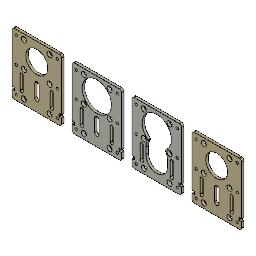
Master Panels v19 (Autodesk Fusion 360 design; units mm, degrees)
Autodesk Fusion 360 part; units mm, degrees
note: some values were not read from the file. Set by a fixed rule: which sketch regions a step uses.
sketch "Sketch1" plane through (0, 0, 0) normal (0, 0, 1) x (1, 0, 0)
  line L0 (-75, 0) -> (75, 0) construction
  line L1 (0, 75) -> (0, -100) construction
  line L2 (0, -100) -> (0, -250) construction
  circle A0 centre (0, 0) radius 12.7
  line L3 (0, 0) -> (-53.033, 53.033) construction
  line L4 (0, 0) -> (75, 0) construction
  circle A1 centre (-15, 15) radius 2.95
  circle A2 centre (15, 15) radius 2.95
  circle A3 centre (-15, -15) radius 2.95
  circle A4 centre (15, -15) radius 2.95
  circle A5 centre (-24, 15) radius 1.4
  circle A6 centre (24, 15) radius 1.4
  circle A7 centre (-24, -15) radius 1.4
  circle A8 centre (24, -15) radius 1.4
  circle A9 centre (-24, -45) radius 1.4
  circle A10 centre (24, -45) radius 1.4
  line L5 (-29, 21) -> (29, 21)
  line L6 (29, 21) -> (29, -51)
  line L7 (29, -51) -> (-29, -51)
  line L8 (-29, -51) -> (-29, 21)
  circle A11 centre (-15, -45) radius 2.95
  circle A12 centre (15, -45) radius 2.95
  line L9 (15.75, -21.7504) -> (15.75, -38.25)
  arc A13 (15.75, -38.25) -> (19.25, -38.25) centre (17.5, -38.25) ccw
  line L10 (19.25, -38.25) -> (19.25, -21.7504)
  arc A14 (19.25, -21.7504) -> (15.75, -21.7504) centre (17.5, -21.7504) ccw
  line L11 (17.5, -20.0004) -> (17.5, -40) construction
  line L12 (-17.5, -20.0004) -> (-17.5, -40) construction
  line L13 (-15.75, -21.7504) -> (-15.75, -38.25)
  arc A15 (-15.75, -21.7504) -> (-19.25, -21.7504) centre (-17.5, -21.7504) ccw
  line L14 (-19.25, -38.25) -> (-19.25, -21.7504)
  arc A16 (-19.25, -38.25) -> (-15.75, -38.25) centre (-17.5, -38.25) ccw
  line L15 (-2.5, -22.5004) -> (-2.5, -37.5)
  arc A17 (-2.5, -37.5) -> (2.5, -37.5) centre (0, -37.5) ccw
  line L16 (2.5, -37.5) -> (2.5, -22.5004)
  arc A18 (2.5, -22.5004) -> (-2.5, -22.5004) centre (0, -22.5004) ccw
  line L17 (0, -20.0004) -> (0, -40) construction
  line L18 (-29, -51) -> (-26, -51)
  line L19 (-26, -51) -> (-26, -39.1)
  line L20 (-26, -39.1) -> (-29, -39.1)
  line L21 (-29, -39.1) -> (-29, -51)
  line L22 (-29, -42) -> (-26, -42)
  line L23 (29, -42) -> (26, -42)
  line L24 (26, -51) -> (26, -39.1)
  line L25 (26, -39.1) -> (29, -39.1)
  dimension "d1" = 25.4
  dimension "d2" = 135
  dimension "d3" = 75
  dimension "d4" = 5.9
  dimension "d5" = 15
  dimension "d8" = 30
  dimension "d9" = -60
  dimension "d10" = 2.8
  dimension "d11" = 9
  dimension "d14" = 48
  dimension "d15" = -60
  dimension "d16" = 5
  dimension "d17" = 6
  dimension "d18" = 5
  dimension "d19" = 6
  dimension "d20" = 3.5
  dimension "d21" = 17.5
  dimension "d22" = 5
  dimension "d38" = 58
  dimension "d39" = 72
  dimension "d42" = 3
  dimension "d43" = 11.9
  dimension "d44" = 9
  measures "d1" diameter of A0
  measures "d2" angle of L3 L4
  measures "d3" distance of A0.centre L3.end
  measures "d4" diameter of A1
  measures "d5" distance of L0 A1.centre
  measures "d10" diameter of A5
  measures "d11" distance of A1.centre A5.centre
  measures "d16" distance of A6.centre L6
  measures "d17" distance of A2.centre L5
  measures "d18" distance of A9.centre L8
  measures "d19" distance of L7 A11.centre
  measures "d20" diameter of A13
  measures "d21" distance of L1 L11
  measures "d22" diameter of A17
  measures "d38" distance of L6.end L7.end
  measures "d39" distance of L5.end L6.end
  measures "d42" distance of L7.end L18.end
  measures "d43" distance of L7.end L20.end
  measures "d44" distance of L7 L22
extrude "Extrude1" add sketch "Sketch1" along normal blind 3 contours L5 L6 L7 L8 L19 L20 L24 L25 | L7 L8 L18 L19 L21 L22 | L6 L7 L23 L24 makes body 1
fillet "Fillet1" radius 2.5 4 edges at (-29, 21, 1.5) (29, 21, 1.5) (29, -51, 1.5) (-29, -51, 1.5) on bodies 1
ref_plane "WorkPlane1" through (0, -15, 3) normal (0, 0, 1) x (1, 0, 0)
sketch "Sketch2" plane through (0, -15, 3) normal (0, 0, 1) x (1, 0, 0)
  arc A0 (-29, -33.5) -> (-26.5, -36) centre (-26.5, -33.5) ccw
  line L0 (-26.5, -36) -> (26.5, -36)
  arc A1 (26.5, -36) -> (29, -33.5) centre (26.5, -33.5) ccw
  line L1 (29, -33.5) -> (29, -27)
  arc A2 (29, 33.5) -> (26.5, 36) centre (26.5, 33.5) ccw
  line L2 (26.5, 36) -> (-26.5, 36)
  arc A3 (-26.5, 36) -> (-29, 33.5) centre (-26.5, 33.5) ccw
  line L3 (-29, 33.5) -> (-29, -24.1)
  arc A4 (19.25, -6.7504) -> (15.75, -6.7504) centre (17.5, -6.7504) ccw
  line L4 (19.25, -6.7504) -> (19.25, -23.25)
  arc A5 (15.75, -23.25) -> (19.25, -23.25) centre (17.5, -23.25) ccw
  line L5 (15.75, -23.25) -> (15.75, -6.7504)
  arc A6 (-15.75, -6.7504) -> (-19.25, -6.7504) centre (-17.5, -6.7504) ccw
  line L6 (-15.75, -6.7504) -> (-15.75, -23.25)
  arc A7 (-19.25, -23.25) -> (-15.75, -23.25) centre (-17.5, -23.25) ccw
  line L7 (-19.25, -23.25) -> (-19.25, -6.7504)
  circle A8 centre (15, -30) radius 2.95
  arc A9 (2.5, -7.5004) -> (-2.5, -7.5004) centre (0, -7.5004) ccw
  line L8 (2.5, -7.5004) -> (2.5, -22.5)
  arc A10 (-2.5, -22.5) -> (2.5, -22.5) centre (0, -22.5) ccw
  line L9 (-2.5, -22.5) -> (-2.5, -7.5004)
  circle A11 centre (24, -30) radius 1.4
  circle A12 centre (-15, -30) radius 2.95
  circle A13 centre (-24, -30) radius 1.4
  circle A14 centre (24, 0) radius 1.4
  circle A15 centre (-24, 0) radius 1.4
  circle A16 centre (24, 30) radius 1.4
  circle A17 centre (-24, 30) radius 1.4
  circle A18 centre (15, 0) radius 2.95
  circle A19 centre (-15, 0) radius 2.95
  circle A20 centre (15, 30) radius 2.95
  circle A21 centre (-15, 30) radius 2.95
  circle A22 centre (0, 15) radius 12.7
  circle A23 centre (0, 15) radius 16.95
  line L10 (29, -27) -> (26, -27)
  line L11 (26, -27) -> (26, -24.1)
  line L12 (26, -24.1) -> (29, -24.1)
  line L13 (29, -24.1) -> (29, 33.5)
  line L14 (-29, -24.1) -> (-26, -24.1)
  line L15 (-26, -24.1) -> (-26, -27)
  line L16 (-26, -27) -> (-29, -27)
  line L17 (-29, -27) -> (-29, -33.5)
  dimension "d27" = 33.9
  measures "d27" diameter of A23
extrude "Extrude2" add sketch "Sketch2" against normal blind 3 separate body contours A0 L0 A1 L1 A2 L2 A3 L3 L10 L11 L12 L13 L14 L15 L16 L17 makes body 2
ref_plane "WorkPlane2" through (0, -15, 3) normal (0, 0, 1) x (1, 0, 0)
sketch "Sketch3" plane through (0, -15, 3) normal (0, 0, 1) x (1, 0, 0)
  arc A0 (-29, -33.5) -> (-26.5, -36) centre (-26.5, -33.5) ccw
  line L0 (-26.5, -36) -> (26.5, -36)
  arc A1 (26.5, -36) -> (29, -33.5) centre (26.5, -33.5) ccw
  line L1 (29, -33.5) -> (29, -27)
  arc A2 (29, 33.5) -> (26.5, 36) centre (26.5, 33.5) ccw
  line L2 (26.5, 36) -> (-26.5, 36)
  arc A3 (-26.5, 36) -> (-29, 33.5) centre (-26.5, 33.5) ccw
  line L3 (-29, 33.5) -> (-29, -24.1)
  arc A4 (19.25, -6.7504) -> (15.75, -6.7504) centre (17.5, -6.7504) ccw
  line L4 (19.25, -6.7504) -> (19.25, -23.25)
  arc A5 (15.75, -23.25) -> (19.25, -23.25) centre (17.5, -23.25) ccw
  line L5 (15.75, -23.25) -> (15.75, -6.7504)
  arc A6 (-15.75, -6.7504) -> (-19.25, -6.7504) centre (-17.5, -6.7504) ccw
  line L6 (-15.75, -6.7504) -> (-15.75, -23.25)
  arc A7 (-19.25, -23.25) -> (-15.75, -23.25) centre (-17.5, -23.25) ccw
  line L7 (-19.25, -23.25) -> (-19.25, -6.7504)
  circle A8 centre (15, -30) radius 2.95
  arc A9 (2.5, -7.5004) -> (-2.5, -7.5004) centre (0, -7.5004) ccw
  line L8 (2.5, -7.5004) -> (2.5, -22.5)
  arc A10 (-2.5, -22.5) -> (2.5, -22.5) centre (0, -22.5) ccw
  line L9 (-2.5, -22.5) -> (-2.5, -7.5004)
  circle A11 centre (24, -30) radius 1.4
  circle A12 centre (-15, -30) radius 2.95
  circle A13 centre (-24, -30) radius 1.4
  circle A14 centre (24, 0) radius 1.4
  circle A15 centre (-24, 0) radius 1.4
  circle A16 centre (24, 30) radius 1.4
  circle A17 centre (-24, 30) radius 1.4
  circle A18 centre (15, 0) radius 2.95
  circle A19 centre (-15, 0) radius 2.95
  circle A20 centre (15, 30) radius 2.95
  circle A21 centre (-15, 30) radius 2.95
  circle A22 centre (0, 15) radius 12.7
  circle A23 centre (0, 15) radius 16.95
  line L10 (12.5, -15) -> (12.5, -7.5004)
  arc A24 (12.5, -7.5004) -> (-12.5, -7.5004) centre (0, -7.5004) ccw
  line L11 (-12.5, -7.5004) -> (-12.5, -15)
  arc A25 (-12.5, -15) -> (12.5, -15) centre (0, -15) ccw
  line L12 (0, -15) -> (0, -7.5004) construction
  line L13 (10, -7.5004) -> (-10, -7.5004)
  line L14 (-10, -7.5004) -> (-10, 7.5004)
  line L15 (-10, 7.5004) -> (10, 7.5004)
  line L16 (10, 7.5004) -> (10, -7.5004)
  line L17 (10, -7.5004) -> (-10, 7.5004) construction
  line L18 (-10, -7.5004) -> (10, 7.5004) construction
  line L19 (29, -27) -> (26, -27)
  line L20 (26, -27) -> (26, -24.1)
  line L21 (26, -24.1) -> (29, -24.1)
  line L22 (29, -24.1) -> (29, 33.5)
  line L23 (-29, -24.1) -> (-26, -24.1)
  line L24 (-26, -24.1) -> (-26, -27)
  line L25 (-26, -27) -> (-29, -27)
  line L26 (-29, -27) -> (-29, -33.5)
  dimension "d31" = 25
  dimension "d32" = 20
  measures "d31" diameter of A24
  measures "d32" distance of L14.end L15.end
extrude "Extrude3" add sketch "Sketch3" against normal blind 3 separate body makes body 3
ref_plane "WorkPlane3" through (0, -15, 3) normal (0, 0, 1) x (1, 0, 0)
sketch "Sketch4" plane through (0, -15, 3) normal (0, 0, 1) x (1, 0, 0)
  arc A0 (-29, -33.5) -> (-26.5, -36) centre (-26.5, -33.5) ccw
  line L0 (-26.5, -36) -> (26.5, -36)
  arc A1 (26.5, -36) -> (29, -33.5) centre (26.5, -33.5) ccw
  line L1 (29, -33.5) -> (29, -27)
  arc A2 (29, 33.5) -> (26.5, 36) centre (26.5, 33.5) ccw
  line L2 (26.5, 36) -> (-26.5, 36)
  arc A3 (-26.5, 36) -> (-29, 33.5) centre (-26.5, 33.5) ccw
  line L3 (-29, 33.5) -> (-29, -24.1)
  arc A4 (19.25, -6.7504) -> (15.75, -6.7504) centre (17.5, -6.7504) ccw
  line L4 (19.25, -6.7504) -> (19.25, -23.25)
  arc A5 (15.75, -23.25) -> (19.25, -23.25) centre (17.5, -23.25) ccw
  line L5 (15.75, -23.25) -> (15.75, -6.7504)
  arc A6 (-15.75, -6.7504) -> (-19.25, -6.7504) centre (-17.5, -6.7504) ccw
  line L6 (-15.75, -6.7504) -> (-15.75, -23.25)
  arc A7 (-19.25, -23.25) -> (-15.75, -23.25) centre (-17.5, -23.25) ccw
  line L7 (-19.25, -23.25) -> (-19.25, -6.7504)
  circle A8 centre (15, -30) radius 2.95
  arc A9 (2.5, -7.5004) -> (-2.5, -7.5004) centre (0, -7.5004) ccw
  line L8 (2.5, -7.5004) -> (2.5, -22.5)
  arc A10 (-2.5, -22.5) -> (2.5, -22.5) centre (0, -22.5) ccw
  line L9 (-2.5, -22.5) -> (-2.5, -7.5004)
  circle A11 centre (24, -30) radius 1.4
  circle A12 centre (-15, -30) radius 2.95
  circle A13 centre (-24, -30) radius 1.4
  circle A14 centre (24, 0) radius 1.4
  circle A15 centre (-24, 0) radius 1.4
  circle A16 centre (24, 30) radius 1.4
  circle A17 centre (-24, 30) radius 1.4
  circle A18 centre (15, 0) radius 2.95
  circle A19 centre (-15, 0) radius 2.95
  circle A20 centre (15, 30) radius 2.95
  circle A21 centre (-15, 30) radius 2.95
  circle A22 centre (0, 15) radius 12.7
  line L10 (29, -27) -> (26, -27)
  line L11 (26, -27) -> (26, -24.1)
  line L12 (26, -24.1) -> (29, -24.1)
  line L13 (29, -24.1) -> (29, 33.5)
  line L14 (-29, -24.1) -> (-26, -24.1)
  line L15 (-26, -24.1) -> (-26, -27)
  line L16 (-26, -27) -> (-29, -27)
  line L17 (-29, -27) -> (-29, -33.5)
extrude "Extrude4" add sketch "Sketch4" against normal blind 3 separate body makes body 4
copy_body "Body->Comp1" bodies 4 removing the originals makes body 5 in component "Component"
copy_body "Body->Comp2" bodies 3 removing the originals makes body 6 in component "Component'"
copy_body "Body->Comp3" bodies 2 removing the originals makes body 7 in component "Component''"
copy_body "Body->Comp4" bodies 1 removing the originals makes body 8 in component "Component'''"
copy_body "Body->Comp1'" bodies 5 removing the originals makes body 9 in component "Component''''"
copy_body "Body->Comp1''" bodies 6 removing the originals makes body 10 in component "Component'''''"
copy_body "Body->Comp1'''" bodies 7 removing the originals makes body 11 in component "Component''''''"
copy_body "Body->Comp1''''" bodies 8 removing the originals makes body 12 in component "Component'''''''"
move_body "Move2" bodies 11 to x (1, 0, 0) y (0, 1, 0) z (0, 0, 1) at (70, 0, 0) in component "Component''''''"
move_body "Move2'" bodies 10 to x (1, 0, 0) y (0, 1, 0) z (0, 0, 1) at (140, 0, 0) in component "Component'''''"
move_body "Move1" bodies 9 to x (1, 0, 0) y (0, 1, 0) z (0, 0, 1) at (210, 0, 0) in component "Component''''"
component "Component" placed x (1, 0, 0) y (0, 1, 0) z (0, 0, 1) at (0, 0, 0)
component "Component'" placed x (1, 0, 0) y (0, 1, 0) z (0, 0, 1) at (0, 0, 0)
component "Component''" placed x (1, 0, 0) y (0, 1, 0) z (0, 0, 1) at (0, 0, 0)
component "Component'''" placed x (1, 0, 0) y (0, 1, 0) z (0, 0, 1) at (0, 0, 0)
component "Component''''" placed x (1, 0, 0) y (0, 1, 0) z (0, 0, 1) at (0, 0, 0) in component "Component"
component "Component'''''" placed x (1, 0, 0) y (0, 1, 0) z (0, 0, 1) at (0, 0, 0) in component "Component'"
component "Component''''''" placed x (1, 0, 0) y (0, 1, 0) z (0, 0, 1) at (0, 0, 0) in component "Component''"
component "Component'''''''" placed x (1, 0, 0) y (0, 1, 0) z (0, 0, 1) at (0, 0, 0) in component "Component'''"
equation "d21 = ( 35 / 2 ) * 1 mm"
equation "d26 = Offset"
equation "d30 = Offset * 2"
equation "d35 = Offset * 3"
equation "Offset = 0 mm"
equation "Spread = 60 mm"
